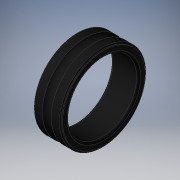
# Autodesk Inventor part: 6007DDU Inner ring
Saved by Autodesk Inventor 2023 (Build 270158000, 158)
## iProperties
Created: 2023-07-20
Part Number: 6007DDU Inner ring
Material: Generic
Catalog Web Link: www.cadenas.de
Description: contact_sealed_type_dd_ddu_IR-NSK
Vendor: NSK_RB
Document SubType Name: Modeling
Designer: psAdmin
Manufacturer: NSK_RB
Mass: 6.75946 g
Surface Area: 44.4129 cm^2
Volume: 6.75946 cm^3
Density: 1 g/cm^3
Appearance: PSOLRGB-128-128-128
Category: PARTsolutions
Company: NSK_RB
PSOL_IDENT_0: {$CADENAS_DATA/23d-libs/nsk_rb/roller_bearings/deep_groove_bb/single_row_dgbb/contact_sealed_type_dd
PSOL_IDENT_1: _ddu_3_ir.prj},201 {VTYP=3D},{NB=6007DDU Inner ring},{LINA=6007DDU Inner ring},{NN=contact_sealed_ty
PSOL_IDENT_2: pe_dd_ddu_IR},{DATE=15.09.2022 00:32:48},{GEOMDATE=18.05.2018 11:36:18},{VERSION=},{LINEID=1980},{WB
PSOL_IDENT_3: VAR=},{WBNUMERIC=}  {NB=6007DDU Inner ring},{LINA=6007DDU Inner ring},{KT=DUMMY},{IDNR=21},{STAN=Sta
PSOL_IDENT_4: ndard},{ORDER=6007DDU},{SD=35},{X=35},{DI1=43.50},{DI2=41.6},{SDE1=54.10},{SDE2=56.00},{D=62},{DD=62
PSOL_IDENT_5: },{B=14},{R=1.0},{CR1=16000},{COR1=10300},{CR2=1630},{COR2=1050},{FO=14.8},{LG=6700},{A=2.08},{BB=1.
PSOL_IDENT_6: 90},{DD1=59.61},{RO=0.60},{RN=0.5},{DD2=67.7},{F=1.70},{DAM1=40.0},{DA1=41.5},{DA2=57.0},{RA=1.0},{D
PSOL_IDENT_7: X=68.5},{CY=3.4},{MASS=0.151},{SC=1}
NB: 6007DDU Inner ring
NN: contact_sealed_type_dd_ddu_IR
NT: NSK
NBSYN: $ORDER. Inner ring
LINA: 6007DDU Inner ring
CATALOG: NSK Rolling Bearing
IDNR: 21
STAN: Standard
ORDER: 6007DDU
SD: 35
X: 35
DI1: 43.5
DI2: 41.6
SDE1: 54.1
SDE2: 56
D: 62
DD: 62
B: 14
R: 1
CR1: 16000
COR1: 10300
CR2: 1630
COR2: 1050
FO: 14.8
LG: 6700
A: 2.08
BB: 1.9
DD1: 59.61
RO: 0.6
RN: 0.5
DD2: 67.7
F: 1.7
DAM1: 40
DA1: 41.5
DA2: 57
RA: 1
DX: 68.5
CY: 3.4
MASS: 0.151
SC: 1
SUPPLIER: NSK_RB
ARTICLENO: 6007DDU Inner ring
BOMINFO: 6007DDU Inner ring
CREATOR: CADENAS GmbH
Title: 6007DDU Inner ring
Author: Cadenas PARTsolutions
Comments: NSK
Autodesk Inventor part; units mm, degrees
sketch "Sketch_1" plane through (0, 0, 0) normal (0, 0, 1) x (1, 0, 0)
  line L0 (14, 0) -> (0, 0)
  arc A0 (0, 18.5) -> (1, 17.5) centre (1, 18.5) ccw
  line L1 (1, 17.5) -> (13, 17.5)
  arc A1 (13, 17.5) -> (14, 18.5) centre (13, 18.5) ccw
  line L2 (14, 18.5) -> (14, 20.8)
  line L3 (14, 20.8) -> (13.356, 20.8)
  line L4 (13.356, 20.8) -> (13.356, 21.75)
  line L5 (13.356, 21.75) -> (9.2673, 21.75)
  arc A2 (4.7327, 21.75) -> (9.2673, 21.75) centre (7, 24.25) ccw
  line L6 (4.7327, 21.75) -> (0.644, 21.75)
  line L7 (0.644, 21.75) -> (0.644, 20.8)
  line L8 (0.644, 20.8) -> (0, 20.8)
  line L9 (0, 20.8) -> (0, 18.5)
  constraints: 20 end point, 6 point on circle, 3 centre point
revolve "Revolution1" add sketch "Sketch_1" angle 360 about axis through (14, 0, 0) along (1, 0, 0)
ref_plane "ip_cst_3_ir_1_1_XY" through (7, 24.25, 0) normal (-1, 0, 0) x (0, 0, -1)
ref_plane "ip_cst_3_ir_1_1_YZ" through (7, 24.25, 0) normal (0, 0, -1) x (0, -1, 0)
ref_plane "ip_cst_3_ir_1_1_ZX" through (7, 24.25, 0) normal (0, -1, 0) x (-1, 0, 0)
ref_plane "ip_cst_3_ir_1_10_XY" through (7, -8.5992, -22.6741) normal (-1, 0, 0) x (0, 0, -1)
ref_plane "ip_cst_3_ir_1_10_YZ" through (7, -8.5992, -22.6741) normal (0, 0, -1) x (0, -1, 0)
ref_plane "ip_cst_3_ir_1_10_ZX" through (7, -8.5992, -22.6741) normal (0, -1, 0) x (-1, 0, 0)
ref_plane "ip_cst_3_ir_1_11_XY" through (7, 2.923, -24.0732) normal (-1, 0, 0) x (0, 0, -1)
ref_plane "ip_cst_3_ir_1_11_YZ" through (7, 2.923, -24.0732) normal (0, 0, -1) x (0, -1, 0)
ref_plane "ip_cst_3_ir_1_11_ZX" through (7, 2.923, -24.0732) normal (0, -1, 0) x (-1, 0, 0)
ref_plane "ip_cst_3_ir_1_12_XY" through (7, 13.7756, -19.9574) normal (-1, 0, 0) x (0, 0, -1)
ref_plane "ip_cst_3_ir_1_12_YZ" through (7, 13.7756, -19.9574) normal (0, 0, -1) x (0, -1, 0)
ref_plane "ip_cst_3_ir_1_12_ZX" through (7, 13.7756, -19.9574) normal (0, -1, 0) x (-1, 0, 0)
ref_plane "ip_cst_3_ir_1_13_XY" through (7, 21.4723, -11.2695) normal (-1, 0, 0) x (0, 0, -1)
ref_plane "ip_cst_3_ir_1_13_YZ" through (7, 21.4723, -11.2695) normal (0, 0, -1) x (0, -1, 0)
ref_plane "ip_cst_3_ir_1_13_ZX" through (7, 21.4723, -11.2695) normal (0, -1, 0) x (-1, 0, 0)
ref_plane "ip_cst_3_ir_1_2_XY" through (7, 21.4723, 11.2695) normal (-1, 0, 0) x (0, 0, -1)
ref_plane "ip_cst_3_ir_1_2_YZ" through (7, 21.4723, 11.2695) normal (0, 0, -1) x (0, -1, 0)
ref_plane "ip_cst_3_ir_1_2_ZX" through (7, 21.4723, 11.2695) normal (0, -1, 0) x (-1, 0, 0)
ref_plane "ip_cst_3_ir_1_3_XY" through (7, 13.7756, 19.9574) normal (-1, 0, 0) x (0, 0, -1)
ref_plane "ip_cst_3_ir_1_3_YZ" through (7, 13.7756, 19.9574) normal (0, 0, -1) x (0, -1, 0)
ref_plane "ip_cst_3_ir_1_3_ZX" through (7, 13.7756, 19.9574) normal (0, -1, 0) x (-1, 0, 0)
ref_plane "ip_cst_3_ir_1_4_XY" through (7, 2.923, 24.0732) normal (-1, 0, 0) x (0, 0, -1)
ref_plane "ip_cst_3_ir_1_4_YZ" through (7, 2.923, 24.0732) normal (0, 0, -1) x (0, -1, 0)
ref_plane "ip_cst_3_ir_1_4_ZX" through (7, 2.923, 24.0732) normal (0, -1, 0) x (-1, 0, 0)
ref_plane "ip_cst_3_ir_1_5_XY" through (7, -8.5992, 22.6741) normal (-1, 0, 0) x (0, 0, -1)
ref_plane "ip_cst_3_ir_1_5_YZ" through (7, -8.5992, 22.6741) normal (0, 0, -1) x (0, -1, 0)
ref_plane "ip_cst_3_ir_1_5_ZX" through (7, -8.5992, 22.6741) normal (0, -1, 0) x (-1, 0, 0)
ref_plane "ip_cst_3_ir_1_6_XY" through (7, -18.1514, 16.0807) normal (-1, 0, 0) x (0, 0, -1)
ref_plane "ip_cst_3_ir_1_6_YZ" through (7, -18.1514, 16.0807) normal (0, 0, -1) x (0, -1, 0)
ref_plane "ip_cst_3_ir_1_6_ZX" through (7, -18.1514, 16.0807) normal (0, -1, 0) x (-1, 0, 0)
ref_plane "ip_cst_3_ir_1_7_XY" through (7, -23.5453, 5.8034) normal (-1, 0, 0) x (0, 0, -1)
ref_plane "ip_cst_3_ir_1_7_YZ" through (7, -23.5453, 5.8034) normal (0, 0, -1) x (0, -1, 0)
ref_plane "ip_cst_3_ir_1_7_ZX" through (7, -23.5453, 5.8034) normal (0, -1, 0) x (-1, 0, 0)
ref_plane "ip_cst_3_ir_1_8_XY" through (7, -23.5453, -5.8034) normal (-1, 0, 0) x (0, 0, -1)
ref_plane "ip_cst_3_ir_1_8_YZ" through (7, -23.5453, -5.8034) normal (0, 0, -1) x (0, -1, 0)
ref_plane "ip_cst_3_ir_1_8_ZX" through (7, -23.5453, -5.8034) normal (0, -1, 0) x (-1, 0, 0)
ref_plane "ip_cst_3_ir_1_9_XY" through (7, -18.1514, -16.0807) normal (-1, 0, 0) x (0, 0, -1)
ref_plane "ip_cst_3_ir_1_9_YZ" through (7, -18.1514, -16.0807) normal (0, 0, -1) x (0, -1, 0)
ref_plane "ip_cst_3_ir_1_9_ZX" through (7, -18.1514, -16.0807) normal (0, -1, 0) x (-1, 0, 0)
ref_plane "ip_cst_3_ir_1a_XY" through (0, 0, 0) normal (1, 0, 0) x (0, 0, -1)
ref_plane "ip_cst_3_ir_1a_YZ" through (0, 0, 0) normal (0, 0, -1) x (0, 1, 0)
ref_plane "ip_cst_3_ir_1a_ZX" through (0, 0, 0) normal (0, 1, 0) x (1, 0, 0)
body "Solid1"
